Autodesk Fusion 360 part; units mm, degrees
(part 3 of 3)
  arc A337 (-108.8447, 47.3677) -> (-108.3447, 46.8677) centre (-108.3447, 47.3677) ccw
  line L341 (-108.8447, 47.3677) -> (-108.8447, 60.3677)
  arc A338 (-108.3447, 60.8677) -> (-108.8447, 60.3677) centre (-108.3447, 60.3677) ccw
  line L342 (-108.3447, 60.8677) -> (-95.3447, 60.8677)
  arc A339 (-94.8447, 60.3677) -> (-95.3447, 60.8677) centre (-95.3447, 60.3677) ccw
  line L343 (-94.8447, 60.3677) -> (-94.8447, 47.3677)
  arc A340 (14.1928, 8.7677) -> (14.6928, 9.2677) centre (14.1928, 9.2677) ccw
  line L344 (14.1928, 8.7677) -> (1.1928, 8.7677)
  arc A341 (0.6928, 9.2677) -> (1.1928, 8.7677) centre (1.1928, 9.2677) ccw
  line L345 (0.6928, 9.2677) -> (0.6928, 22.2677)
  arc A342 (1.1928, 22.7677) -> (0.6928, 22.2677) centre (1.1928, 22.2677) ccw
  line L346 (1.1928, 22.7677) -> (14.1928, 22.7677)
  arc A343 (14.6928, 22.2677) -> (14.1928, 22.7677) centre (14.1928, 22.2677) ccw
  line L347 (14.6928, 22.2677) -> (14.6928, 9.2677)
  arc A344 (-47.7197, 65.9177) -> (-47.2197, 66.4177) centre (-47.7197, 66.4177) ccw
  line L348 (-47.7197, 65.9177) -> (-60.7197, 65.9177)
  arc A345 (-61.2197, 66.4177) -> (-60.7197, 65.9177) centre (-60.7197, 66.4177) ccw
  line L349 (-61.2197, 66.4177) -> (-61.2197, 79.4177)
  arc A346 (-60.7197, 79.9177) -> (-61.2197, 79.4177) centre (-60.7197, 79.4177) ccw
  line L350 (-60.7197, 79.9177) -> (-47.7197, 79.9177)
  arc A347 (-47.2197, 79.4177) -> (-47.7197, 79.9177) centre (-47.7197, 79.4177) ccw
  line L351 (-47.2197, 79.4177) -> (-47.2197, 66.4177)
  arc A348 (-9.6197, 65.9177) -> (-9.1197, 66.4177) centre (-9.6197, 66.4177) ccw
  line L352 (-9.6197, 65.9177) -> (-22.6197, 65.9177)
  arc A349 (-23.1197, 66.4177) -> (-22.6197, 65.9177) centre (-22.6197, 66.4177) ccw
  line L353 (-23.1197, 66.4177) -> (-23.1197, 79.4177)
  arc A350 (-22.6197, 79.9177) -> (-23.1197, 79.4177) centre (-22.6197, 79.4177) ccw
  line L354 (-22.6197, 79.9177) -> (-9.6197, 79.9177)
  arc A351 (-9.1197, 79.4177) -> (-9.6197, 79.9177) centre (-9.6197, 79.4177) ccw
  line L355 (-9.1197, 79.4177) -> (-9.1197, 66.4177)
  arc A352 (-85.8197, 65.9177) -> (-85.3197, 66.4177) centre (-85.8197, 66.4177) ccw
  line L356 (-85.8197, 65.9177) -> (-98.8197, 65.9177)
  arc A353 (-99.3197, 66.4177) -> (-98.8197, 65.9177) centre (-98.8197, 66.4177) ccw
  line L357 (-99.3197, 66.4177) -> (-99.3197, 79.4177)
  arc A354 (-98.8197, 79.9177) -> (-99.3197, 79.4177) centre (-98.8197, 79.4177) ccw
  line L358 (-98.8197, 79.9177) -> (-85.8197, 79.9177)
  arc A355 (-85.3197, 79.4177) -> (-85.8197, 79.9177) centre (-85.8197, 79.4177) ccw
  line L359 (-85.3197, 79.4177) -> (-85.3197, 66.4177)
  arc A356 (-38.1947, 46.8677) -> (-37.6947, 47.3677) centre (-38.1947, 47.3677) ccw
  line L360 (-38.1947, 46.8677) -> (-51.1947, 46.8677)
  arc A357 (-51.6947, 47.3677) -> (-51.1947, 46.8677) centre (-51.1947, 47.3677) ccw
  line L361 (-51.6947, 47.3677) -> (-51.6947, 60.3677)
  arc A358 (-51.1947, 60.8677) -> (-51.6947, 60.3677) centre (-51.1947, 60.3677) ccw
  line L362 (-51.1947, 60.8677) -> (-38.1947, 60.8677)
  arc A359 (-37.6947, 60.3677) -> (-38.1947, 60.8677) centre (-38.1947, 60.3677) ccw
  line L363 (-37.6947, 60.3677) -> (-37.6947, 47.3677)
  arc A360 (-176.3072, 84.9677) -> (-175.8072, 85.4677) centre (-176.3072, 85.4677) ccw
  line L364 (-176.3072, 84.9677) -> (-189.3072, 84.9677)
  arc A361 (-189.8072, 85.4677) -> (-189.3072, 84.9677) centre (-189.3072, 85.4677) ccw
  line L365 (-189.8072, 85.4677) -> (-189.8072, 98.4677)
  arc A362 (-189.3072, 98.9677) -> (-189.8072, 98.4677) centre (-189.3072, 98.4677) ccw
  line L366 (-189.3072, 98.9677) -> (-176.3072, 98.9677)
  arc A363 (-175.8072, 98.4677) -> (-176.3072, 98.9677) centre (-176.3072, 98.4677) ccw
  line L367 (-175.8072, 98.4677) -> (-175.8072, 85.4677)
  arc A364 (-84.5509, 85.9677) -> (-84.0509, 86.4677) centre (-84.5509, 86.4677) ccw
  line L368 (-84.5509, 85.9677) -> (-90.5509, 85.9677)
  arc A365 (-91.0509, 86.4677) -> (-90.5509, 85.9677) centre (-90.5509, 86.4677) ccw
  line L369 (-91.0509, 86.4677) -> (-91.0509, 100.4677)
  arc A366 (-90.5509, 100.9677) -> (-91.0509, 100.4677) centre (-90.5509, 100.4677) ccw
  line L370 (-90.5509, 100.9677) -> (-84.5509, 100.9677)
  arc A367 (-84.0509, 100.4677) -> (-84.5509, 100.9677) centre (-84.5509, 100.4677) ccw
  line L371 (-84.0509, 100.4677) -> (-84.0509, 86.4677)
  circle A368 centre (107.7226, -51.4273) radius 1.75
  circle A369 centre (107.7226, 112.8427) radius 1.75
  circle A370 centre (-222.9474, 112.8427) radius 1.75
  circle A371 centre (-222.9474, -51.4273) radius 1.75
  line L372 (40, -20) -> (113.7226, -20)
  line L373 (113.7226, -20) -> (113.7226, -47.2306)
  line L374 (113.7226, -47.2306) -> (40, -47.2306)
  line L375 (40, -47.2306) -> (40, -20)
  dimension "d5" = 3.5
  dimension "d6" = 6
  dimension "d7" = 6
  dimension "d10" = 3.5
  dimension "d11" = 6
  dimension "d12" = 6
  dimension "d13" = 3.5
  dimension "d14" = 6
  dimension "d15" = 6
  dimension "d16" = 3.5
  dimension "d17" = 6
  dimension "d18" = 6
  constraint horizontal L372
  constraint vertical L373
  constraint horizontal L374
  constraint vertical L375
  constraint coincident L170 L373.end
  measures "d5" diameter of A368
  measures "d6" distance of L169 A368.centre
  measures "d7" distance of L170 A368.centre
  measures "d10" diameter of A369
  measures "d11" distance of L171 A369.centre
  measures "d12" distance of L170 A369.centre
  measures "d13" diameter of A370
  measures "d14" distance of L168 A370.centre
  measures "d15" distance of L171 A370.centre
  measures "d16" diameter of A371
  measures "d17" distance of L168 A371.centre
  measures "d18" distance of L169 A371.centre
fillet "Fillet1" radius 9 4 edges at (-113.7226, 57.4273, 1.25) (-113.7226, -118.8427, 1.25) (228.9474, -118.8427, 1.25) (228.9474, 57.4273, 1.25)
extrude "Extrude2" cut sketch "Sketch3" against normal blind 30 contours L170 L372 L373 L374 L375 | A368 | A369 | A370 | A371
